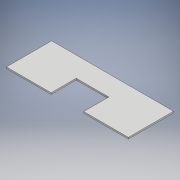
# Autodesk Inventor part: PCB
Saved by Autodesk Inventor 2018 (Build 220112000, 112)
## iProperties
Created: 2018-05-12
Part Number: PCB
Material: Generic
Document SubType Name: Modeling
Designer: Mandus
Density: 1 g/cm^3
Appearance: Default
Author: Mandus
Autodesk Inventor part; units mm, degrees
ref_plane "YZ Plane" through (0, 0, 0) normal (1, 0, 0) x (0, 1, 0)
ref_plane "XZ Plane" through (0, 0, 0) normal (0, 1, 0) x (-1, 0, 0)
ref_plane "XY Plane" through (0, 0, 0) normal (0, 0, 1) x (1, 0, 0)
sketch "Sketch1" plane through (0, 0, 0) normal (0, 0, 1) x (1, 0, 0)
  line L0 (0, 0) -> (44.5, 0)
  line L1 (44.5, 0) -> (44.5, 45)
  line L2 (44.5, 45) -> (0, 45)
  line L3 (0, 45) -> (0, 0)
  line L4 (44.5, 45) -> (77, 45)
  line L5 (77, 45) -> (77, 25)
  line L6 (77, 25) -> (44.5, 25)
  line L7 (44.5, 25) -> (44.5, 45)
  line L8 (77, 45) -> (121.5, 45)
  line L9 (121.5, 45) -> (121.5, 0)
  line L10 (121.5, 0) -> (77, 0)
  line L11 (77, 0) -> (77, 45)
  dimension "d11" = 44.5
  dimension "d12" = 45
  dimension "d13" = 32.5
  dimension "d14" = 20
  dimension "d15" = 44.5
  dimension "d16" = 45
  constraints: 24 end point, 6 parallel, 3 horizontal, 3 perpendicular
  measures "d11" distance of L2.end L1.end
  measures "d12" distance of L1.end L0.end
  measures "d13" distance of L5.end L6.end
  measures "d14" distance of L4.end L5.end
  measures "d15" distance of L9.end L10.end
  measures "d16" distance of L8.end L9.end
extrude "Extrusion1" add sketch "Sketch1" along normal blind 1.6
body "Solid1"
